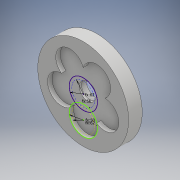
# Autodesk Inventor part: TERMINAL-GEAR-BASE
Saved by Autodesk Inventor 2018 (Build 220112000, 112)
## iProperties
Created: 2026-09-04
Part Number: TERMINAL-GEAR-BASE
Material: Generic
Document SubType Name: Modeling
Designer: neo
Density: 1 g/cm^3
Appearance: Default
Author: neo
Autodesk Inventor part; units mm, degrees
ref_plane "YZ Plane" through (0, 0, 0) normal (1, 0, 0) x (0, 1, 0)
ref_plane "XZ Plane" through (0, 0, 0) normal (0, 1, 0) x (-1, 0, 0)
ref_plane "XY Plane" through (0, 0, 0) normal (0, 0, 1) x (1, 0, 0)
sketch "Sketch1" plane through (0, 0, 0) normal (0, 1, 0) x (-1, 0, 0)
  circle A0 centre (0, 0) radius 10 construction
  circle A1 centre (0, 0) radius 23.5
  circle A2 centre (0, 0) radius 100
  circle A3 centre (0, 0) radius 18.5
  dimension "d0" = 20
  dimension "d1" = 47
  dimension "d2" = 200
  dimension "d3" = 37
  constraints: 4 centre point, 4 coincident
  measures "d0" diameter of A0
  measures "d1" diameter of A1
  measures "d2" diameter of A2
  measures "d3" diameter of A3
extrude "Extrusion1" add sketch "Sketch1" along normal blind 30 contours A2
extrude "Extrusion2" add sketch "Sketch1" along normal blind 15 contours A1
sketch "Sketch2" plane through (0, 0, 0) normal (0, -1, 0) x (1, 0, 0)
  circle A0 centre (0, 0) radius 25 construction
  circle A1 centre (0, -50) radius 25 construction
  circle A2 centre (0, 0) radius 31
  circle A3 centre (0, -50) radius 31
  dimension "dp" = 50
  dimension "d9" = 50
  dimension "d10" = 62
  dimension "d11" = 62
  constraints: 4 centre point, 3 coincident, 1 equal radius
  measures "dp" diameter of A0
  measures "d9" diameter of A1
  measures "d10" diameter of A2
  measures "d11" diameter of A3
extrude "Extrusion3" cut sketch "Sketch2" against normal blind 10 contours A2 A3 | A3 A2 picked at (0.2237, 14.1835) picked at (-2.1631, -26.7711)
extrude "Extrusion4" cut sketch "Sketch2" against normal blind 10 contours A3 A2 | A2 A3 picked at (-2.1631, -26.7711) picked at (0.2237, -64.1835)
pattern_circular "Circular Pattern1" count 5 over 360 about axis through (0, 0, 0) along (0, 1, 0) of "Extrusion4"
equation "\"d9\" = dp"
equation "\"d11\" = d10"
equation "\"d14\" = d12"
equation "\"modul\" = 2"
equation "\"d12\" = 10"
body "Solid1"
